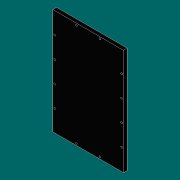
# Autodesk Inventor part: back
Saved by Autodesk Inventor 2016 (Build 200138000, 138)
## iProperties
Created: 2015-10-05
Part Number: back
Material: ABS Plastic
Document SubType Name: Modeling
Designer: Sawaiz
Density: 1.06 g/cm^3
Appearance: Smooth - Black
Author: Sawaiz
Autodesk Inventor part; units mm, degrees
ref_plane "YZ Plane" through (0, 0, 0) normal (1, 0, 0) x (0, 1, 0)
ref_plane "XZ Plane" through (0, 0, 0) normal (0, 1, 0) x (-1, 0, 0)
ref_plane "XY Plane" through (0, 0, 0) normal (0, 0, 1) x (1, 0, 0)
sketch "Sketch1" plane through (0, 0, 0) normal (0, 1, 0) x (-1, 0, 0)
  line L0 (60, -90) -> (-60, -90)
  line L1 (-60, -90) -> (-60, 90)
  line L2 (-60, 90) -> (60, 90)
  line L3 (60, 90) -> (60, -90)
  line L4 (60, -90) -> (-60, 90) construction
  line L5 (-60, -90) -> (60, 90) construction
  point P0 (0, 0)
  dimension "d0" = 120
  dimension "d1" = 180
  constraints: 12 end point, 2 midpoint, 2 parallel, 1 horizontal, 1 perpendicular
  measures "d0" distance of L1.end L2.end
  measures "d1" distance of L0.end L1.end
extrude "Extrusion1" add sketch "Sketch1" along normal blind 6.35
sketch "Sketch2" plane through (0, 6.35, 0) normal (0, 1, 0) x (1, 0, 0)
  line L0 (56.825, -54) -> (56.825, -18)
  line L1 (56.825, -18) -> (56.825, 18)
  line L2 (56.825, 18) -> (56.825, 54)
  line L3 (56.825, 54) -> (-56.825, 54)
  line L4 (-56.825, -54) -> (56.825, -54)
  line L5 (56.825, -18) -> (-56.825, -18)
  line L6 (-56.825, 18) -> (56.825, 18)
  line L7 (20, 86.825) -> (-20, 86.825)
  line L8 (-20, 86.825) -> (-20, -86.825)
  line L9 (20, -86.825) -> (20, 86.825)
  line L10 (60, 90) -> (-60, 90) projected
  line L11 (-60, 90) -> (-60, -90) projected
  line L12 (-60, -90) -> (60, -90) projected
  line L13 (60, -90) -> (60, 90) projected
  line L14 (-56.825, 54) -> (-56.825, 18)
  line L15 (-56.825, -18) -> (-56.825, 18)
  line L16 (-56.825, -18) -> (-56.825, -54)
  line L17 (20, -86.825) -> (-20, -86.825)
  point P0 (0, 0)
  dimension "d7" = 3.175
  dimension "d15" = 40
  dimension "d16" = 36
  dimension "d18" = 40
  dimension "d19" = 36
  dimension "d20" = 3.175
  dimension "d21" = 3.175
  dimension "d22" = 3.175
  constraints: 29 end point, 5 equal length, 4 point on line, 3 horizontal, 3 vertical, 2 collinear, 2 perpendicular
  measures "d7" distance between parallel lines of L10 L7
  measures "d15" distance between parallel lines of L13 L9
  measures "d16" distance from line of L12 L0.start
  measures "d18" distance of L9.start L8.end
  measures "d19" distance of L0.start L0.end
  measures "d20" distance between parallel lines of L11 L16
  measures "d21" distance between parallel lines of L12 L17
  measures "d22" distance between parallel lines of L13 L2
hole "Hole1" at (20, 6.35, 86.825) at (-20, 6.35, 86.825) at (-20, 6.35, -86.825) at (20, 6.35, -86.825) at (56.825, 6.35, -54) at (56.825, 6.35, 18) at (56.825, 6.35, -18) at (-56.825, 6.35, -18) at (-56.825, 6.35, 18) at (-56.825, 6.35, 54) at (-56.825, 6.35, -54) at (56.825, 6.35, 54) direction (0, -1, 0) diameter 3 end through all
equation "\"d0\" = width"
equation "\"d1\" = height"
equation "\"d2\" = materialThickness"
equation "\"d7\" = 0.5 * materialThickness"
equation "\"d15\" = 0.333333 * width"
equation "\"d16\" = 0.2 * height"
equation "\"d18\" = 0.333333 * width"
equation "\"d19\" = 0.2 * height"
equation "\"d20\" = 0.5 * materialThickness"
equation "\"d21\" = 0.5 * materialThickness"
equation "\"d22\" = 0.5 * materialThickness"
equation "\"height\" = 180"
equation "\"width\" = 120"
equation "\"depth\" = 115"
equation "\"materialThickness\" = 6.35"
equation "\"laserKerf\" = 0.1"
equation "\"cardPinDiameter\" = 3"
equation "\"spoolDiameter\" = 95"
equation "\"cardFillet\" = 2.88"
equation "\"cardSelected\" = 1"
equation "\"cardHeight\" = 53.98"
equation "\"cardThickness\" = 0.76"
equation "\"cardWidth\" = 85.6"
equation "\"centeralShaftDiameter\" = 8"
equation "\"cardClearence\" = 0.5"
equation "\"bearingWidth\" = 8"
equation "\"bearingOd\" = 22"
equation "\"axleHeight\" = 95"
equation "\"nutTrapwidth\" = 5.5"
equation "\"nutTrapDepth\" = 2.5"
equation "\"nutTrapClearence\" = 2"
body "Solid1"
